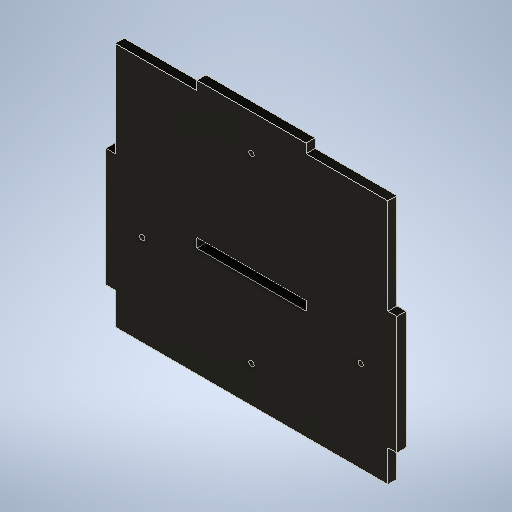
# Autodesk Inventor part: back
Saved by Autodesk Inventor 2025.3 (Build 293356030, 356C)
## iProperties
Created: 2026-06-26
Part Number: back
Material: ABS Plastic
Document SubType Name: Modeling
Designer: user
Density: 1.06 g/cm^3
Appearance: Gunmetal
Author: user
Autodesk Inventor part; units mm, degrees
ref_plane "YZ Plane" through (0, 0, 0) normal (1, 0, 0) x (0, 1, 0)
ref_plane "XZ Plane" through (0, 0, 0) normal (0, 1, 0) x (-1, 0, 0)
ref_plane "XY Plane" through (0, 0, 0) normal (0, 0, 1) x (1, 0, 0)
sketch "Sketch1" plane through (0, 0, 0) normal (0, 0, 1) x (1, 0, 0)
  line L0 (0, 0) -> (150, 0)
  line L1 (150, 0) -> (150, 135)
  line L2 (150, 135) -> (0, 135)
  line L3 (0, 135) -> (0, 0)
  line L4 (0, 17.5) -> (-5, 17.5)
  line L5 (-5, 17.5) -> (-5, 82.5)
  line L6 (-5, 82.5) -> (0, 82.5)
  line L7 (0, 82.5) -> (0, 17.5)
  line L8 (75, 0) -> (75, 135) construction
  line L9 (150, 17.5) -> (155, 17.5)
  line L10 (155, 17.5) -> (155, 82.5)
  line L11 (155, 82.5) -> (150, 82.5)
  line L12 (150, 82.5) -> (150, 17.5)
  line L13 (45, 60) -> (105, 60)
  line L14 (105, 60) -> (105, 65)
  line L15 (105, 65) -> (45, 65)
  line L16 (45, 65) -> (45, 60)
  line L17 (0, 50) -> (150, 50) construction
  line L18 (45, 135) -> (105, 135)
  line L19 (105, 135) -> (105, 140)
  line L20 (105, 140) -> (45, 140)
  line L21 (45, 140) -> (45, 135)
  point P0 (150, 17.5)
  point P1 (150, 82.5)
  point P2 (0, 82.5)
  point P3 (10, 0)
  point P4 (45, 62.5)
  dimension "d0" = 150
  dimension "d1" = 135
  dimension "d2" = 5
  dimension "d3" = 65
  dimension "d6" = 60
  dimension "d7" = 5
  dimension "d14" = 30
  dimension "d30" = 60
  dimension "d31" = 5
  dimension "d32" = 45
  dimension "d58" = 52.5
  dimension "d59" = 60
  constraints: 44 end point, 8 parallel, 5 midpoint, 4 horizontal, 4 perpendicular, 4 symmetric about line, 3 point on line
  measures "d0" distance of L2.end L1.end
  measures "d1" distance of L1.end L0.end
  measures "d2" distance of L5.end L6.end
  measures "d3" distance of L4.end L5.end
  measures "d6" distance of L15.end L14.end
  measures "d7" distance of L14.end L13.end
  measures "d14" distance from line of point (45, 62.5) L8
  measures "d30" distance of L20.end L19.end
  measures "d31" distance of L19.end L18.end
  measures "d32" distance between parallel lines of L1 L19
  measures "d58" distance between parallel lines of L2 L6
  measures "d59" distance between parallel lines of L0 L13
extrude "Extrusion1" add sketch "Sketch1" along normal blind 5
sketch "Sketch2" plane through (0, 0, 5) normal (0, 0, 1) x (1, 0, 0)
  line L0 (150, 135) -> (0, 135) projected
  line L1 (0, 0) -> (150, 0) projected
  line L2 (0, 135) -> (0, 82.5) projected
  line L3 (0, 17.5) -> (0, 0) projected
  point P0 (75, 20)
  dimension "d24" = 20
  dimension "d29" = 75
  measures "d24" distance from line of L1 point (75, 20)
  measures "d29" distance from line of L3 point (75, 20)
hole "Hole1" at (75, 20, 5) direction (0, 0, -1) diameter 3 end through all
sketch "Sketch3" plane through (0, 0, 5) normal (0, 0, 1) x (1, 0, 0)
  line L0 (105, 140) -> (45, 140) projected
  line L1 (45, 140) -> (45, 135) projected
  line L2 (0, 135) -> (0, 82.5) projected
  point P0 (0, 0)
  point P1 (75, 120)
  dimension "d40" = 20
  dimension "d45" = 75
  measures "d40" distance from line of point (75, 120) L0
  measures "d45" distance from line of L2 point (75, 120)
hole "Hole2" at (75, 120, 5) direction (0, 0, -1) diameter 3 end through all
sketch "Sketch4" plane through (0, 0, 5) normal (0, 0, 1) x (1, 0, 0)
  line L0 (-5, 82.5) -> (-5, 17.5) projected
  line L1 (0, 82.5) -> (-5, 82.5) projected
  line L2 (155, 82.5) -> (150, 82.5) projected
  line L3 (155, 17.5) -> (155, 82.5) projected
  point P0 (0, 0)
  point P1 (135, 50)
  point P2 (15, 50)
  point P3 (-5, 50)
  point P4 (-2.5, 82.5)
  dimension "d54" = 20
  dimension "d55" = 32.5
  dimension "d56" = 32.5
  dimension "d57" = 20
  constraints: 2 midpoint
  measures "d54" distance of point (-5, 50) point (15, 50)
  measures "d55" vertical distance of point (15, 50) point (-2.5, 82.5)
  measures "d56" distance from line of point (135, 50) L2
  measures "d57" distance from line of L3 point (135, 50)
hole "Hole3" at (135, 50, 5) at (15, 50, 5) direction (0, 0, -1) diameter 3 end through all
body "Solid1"
